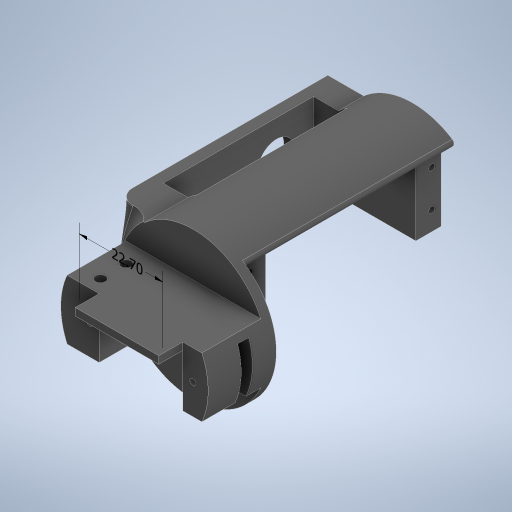
# Autodesk Inventor part: arm_2
Saved by Autodesk Inventor 2024.1 (Build 281209000, 209)
## iProperties
Created: 2025-01-27
Part Number: arm_2
Material: 一般
Document SubType Name: Modeling
Designer: hibik
Density: 1 g/cm^3
Appearance: 既定
Author: hibik
Autodesk Inventor part; units mm, degrees
sketch "スケッチ1" plane through (0, 0, 0) normal (0, 1, 0) x (-1, 0, 0)
  line L0 (11.35, 0) -> (-11.35, 0)
  line L1 (-11.35, 0) -> (-11.35, -25)
  line L2 (-11.35, -25) -> (11.35, -25)
  line L3 (11.35, -25) -> (11.35, 0)
  point P0 (0, 0)
  point P1 (0, 0)
  dimension "d0" = 22.7
  dimension "d9" = 25
  constraints: 8 end point, 2 parallel, 1 coincident, 1 horizontal, 1 midpoint, 1 perpendicular
  measures "d0" distance of L0.start L0.end
  measures "d9" distance of L2.end L0.start
extrude "押し出し1" add sketch "スケッチ1" along normal blind 2
ref_plane "作業平面1" through (-11.35, 0, -22.5) normal (0, 0, 1) x (1, 0, 0)
sketch "スケッチ2" plane through (-11.35, 0, -22.5) normal (0, 0, 1) x (1, 0, 0)
  line L0 (0, 0) -> (0, 2) projected
  line L1 (0, 0) -> (22.7, 0)
  line L2 (22.7, 0) -> (22.7, -12.2)
  line L3 (22.7, -12.2) -> (0, -12.2)
  line L4 (0, -12.2) -> (0, 0)
  line L5 (22.7, 0) -> (22.7, 2) projected
  line L6 (0, -12.2) -> (22.7, -12.2)
  line L7 (22.7, -12.2) -> (22.7, -14.2)
  line L8 (22.7, -14.2) -> (0, -14.2)
  line L9 (0, -14.2) -> (0, -12.2)
  circle A0 centre (9.6, -6.1) radius 20
  line L10 (0, -14.2) -> (-8.6863, -14.2)
  line L11 (-8.6863, -14.2) -> (-8.6863, 2)
  line L12 (-8.6863, 2) -> (0, 2)
  line L13 (0, 2) -> (0, -14.2)
  line L14 (22.7, -14.2) -> (27.8863, -14.2)
  line L15 (27.8863, -14.2) -> (27.8863, 2)
  line L16 (27.8863, 2) -> (22.7, 2)
  line L17 (22.7, 2) -> (22.7, -14.2)
  circle A1 centre (9.6, -6.1) radius 17.5 construction
  circle A2 centre (16.6, -6.1) radius 10.5 construction
  circle A3 centre (16.6, -6.1) radius 6.1
  line L18 (0, 0) -> (22.7, 0) projected
  point P0 (11.35, 0)
  point P1 (22.7, 0)
  dimension "d4" = 12.2
  dimension "d5" = 2
  dimension "d6" = 40
  dimension "d32" = 35
  dimension "d33" = 21
  constraints: 32 end point, 8 parallel, 4 centre point, 4 horizontal, 4 perpendicular, 4 point on circle, 4 tangent, 2 coincident, 2 collinear, 1 horizontal alignment
  measures "d4" distance of L1.end L2.end
  measures "d5" distance of L6.end L7.end
  measures "d6" diameter of A0
  measures "d32" diameter of A1
  measures "d33" diameter of A2
extrude "押し出し2" add sketch "スケッチ2" against normal blind 2.5
ref_plane "作業平面3" through (11.35, 0, -25) normal (0, 0, -1) x (-1, 0, 0)
sketch "スケッチ4" plane through (11.35, 0, -25) normal (0, 0, -1) x (-1, 0, 0)
  line L0 (-0.1288, 8.9) -> (26.3288, 8.9)
  circle A0 centre (13.1, -6.1) radius 20 projected
  line L1 (22.7, 2) -> (0, 2) projected
  dimension "d40" = 15
  constraints: 2 end point, 2 point on circle, 1 horizontal
  measures "d40" distance from line of A0.centre L0
extrude "押し出し4" add sketch "スケッチ4" along normal blind 57 contours A0 L0 picked at (10.0107, 9.8077)
ref_plane "作業平面2" through (7.9, 0, -25) normal (1, 0, 0) x (0, 0, -1)
extrude "押し出し7" add sketch "スケッチ2" along normal blind 16 contours L4 L9 L10 L11 L12 L0 | L11 A0 | L5 L16 L15 L14 L7 L2 | A0 L15
sketch "スケッチ7" plane through (11.35, -14.2, -22.5) normal (0, -1, 0) x (1, 0, 0)
  line L0 (0, 16) -> (0, 0) projected
  line L1 (0, 4) -> (19.8753, 4)
  line L2 (19.8753, 4) -> (19.8753, 7)
  line L3 (19.8753, 7) -> (0, 7)
  line L4 (0, 7) -> (0, 4)
  line L5 (5.1863, 0) -> (-31.3863, 0) projected
  point P0 (-11.35, 22.5)
  point P1 (0, 7)
  dimension "d28" = 4
  dimension "d29" = 3
  constraints: 8 end point, 2 parallel, 1 horizontal, 1 perpendicular, 1 point on line
  measures "d28" distance between parallel lines of L5 L1
  measures "d29" distance of L1.end L2.end
extrude "押し出し8" cut sketch "スケッチ7" against normal up to surface (14.2 mm away)
sketch "スケッチ9" plane through (0, 2, 0) normal (0, 1, 0) x (1, 0, 0)
  circle A0 centre (-14.6932, 17.2) radius 1.6 projected
  circle A1 centre (-14.6932, 10.2) radius 1.6 projected
  circle A2 centre (-14.6932, 17.2) radius 1.35
  circle A3 centre (-14.6932, 10.2) radius 1.35
  point P0 (0, 0)
  dimension "d34" = 2.7
  dimension "d35" = 2.7
  constraints: 2 centre point, 2 coincident
  measures "d34" diameter of A2
  measures "d35" diameter of A3
extrude "押し出し9" cut sketch "スケッチ9" against normal through all contours A2 | A3
ref_plane "作業平面6" through (6.05, -6.1, -22.5) normal (1, 0, 0) x (0, 0, -1)
ref_plane "作業平面5" through (-1.75, -6.1, -22.5) normal (1, 0, 0) x (0, 0, -1)
sketch "スケッチ10" plane through (6.05, -6.1, -22.5) normal (1, 0, 0) x (0, 0, -1)
  line L0 (2.5, 15) -> (59.5, 15) projected
  line L1 (59.5, 15) -> (52.6, 15)
  line L2 (52.6, 15) -> (52.6, -5.1)
  line L3 (52.6, -5.1) -> (59.5, -5.1)
  line L4 (59.5, -5.1) -> (59.5, 15)
  line L5 (2.5, -20) -> (2.5, 15) projected
  line L6 (11.8, 15) -> (2.5, 15)
  line L7 (2.5, 15) -> (2.5, -5.1)
  line L8 (2.5, -5.1) -> (11.8, -5.1)
  line L9 (11.8, -5.1) -> (11.8, 15)
  point P0 (-22.5, 6.1)
  dimension "d43" = 20.1
  dimension "d44" = 40.8
  dimension "d45" = 6.9
  constraints: 16 end point, 4 parallel, 2 horizontal, 2 perpendicular, 2 point on line, 1 collinear
  measures "d43" distance of L3.end L0.end
  measures "d44" distance between parallel lines of L2 L9
  measures "d45" distance of L2.end L3.end
extrude "押し出し10" add sketch "スケッチ10" against normal up to surface round surface about axis through (-1.75, -6.1, -22.5) along (0, 0, -1) radius 20 far side no
fillet "フィレット1" radius 1 2 edges at (11.4788, 8.9, -53.5) (-14.9788, 8.9, -54.7)
ref_plane "作業平面8" through (-24.75, -6.1, -22.5) normal (1, 0, 0) x (0, 0, -1)
ref_plane "作業平面7" through (-26.75, -6.1, -22.5) normal (1, 0, 0) x (0, 0, -1)
sketch "スケッチ11" plane through (-24.75, -6.1, -22.5) normal (1, 0, 0) x (0, 0, -1)
  line L0 (2.5, -20) -> (2.5, 16.8421) projected
  line L1 (59.5, -5.1) -> (59.5, 20) projected
  line L2 (52.6, -5.1) -> (59.5, -5.1) projected
  line L3 (2.5, -5.1) -> (11.8, -5.1) projected
  line L4 (11.8, 15) -> (52.6, 15) projected
  line L5 (59.5, -5.1) -> (2.5, -5.1)
  line L6 (2.5, -5.1) -> (2.5, 15)
  line L7 (2.5, 15) -> (59.5, 15)
  line L8 (59.5, 15) -> (59.5, -5.1)
  point P0 (-22.5, 6.1)
  point P1 (59.5, 16.8421)
  point P2 (59.5, 15)
  constraints: 8 end point, 2 parallel, 1 collinear, 1 horizontal, 1 perpendicular, 1 point on line
extrude "押し出し11" add sketch "スケッチ11" along normal blind 3
sketch "スケッチ12" plane through (-21.75, -6.1, -22.5) normal (1, 0, 0) x (0, 0, -1)
  line L0 (11.8, -5.1) -> (11.8, 15) projected
  line L1 (52.6, 15) -> (52.6, -5.1) projected
  line L2 (59.5, -5.1) -> (59.5, 15) projected
  line L3 (2.5, -20) -> (2.5, 16.8421) projected
  line L4 (59.5, 15) -> (2.5, 15) projected
  line L5 (59.5, -5.1) -> (59.5, 15) projected
  line L6 (2.5, -5.1) -> (59.5, -5.1) projected
  line L7 (2.5, 15) -> (2.5, -5.1) projected
  point P0 (-22.5, 6.1)
  point P1 (11.8, 15)
  point P2 (2.5, 15)
  point P3 (59.5, 15)
extrude "押し出し12" add sketch "スケッチ12" along normal up to surface contours L6 L3 L4 L0 | L1 L4 L2 L6 round surface about axis through (-1.75, -6.1, -22.5) along (0, 0, -1) radius 20 far side no
sketch "スケッチ13" plane through (-24.75, -6.1, -22.5) normal (-1, 0, 0) x (0, 0, 1)
  circle A0 centre (-42.55, 4.95) radius 10.05
  line L0 (-52.6, 15) -> (-11.8, 15) projected
  line L1 (-2.5, -5.1) -> (-59.5, -5.1) projected
  line L2 (-52.6, -5.1) -> (-52.6, 15) projected
  line L3 (-52.6, 15) -> (-52.6, -5.1) projected
  circle A1 centre (-42.55, 4.95) radius 5
  line L4 (-52.6, 16.8421) -> (-52.6, 15) projected
  line L5 (-52.6, 16.8421) -> (-52.6, 15) projected
  point P0 (22.5, 6.1)
  dimension "d55" = 10
  constraints: 3 tangent, 2 centre point, 1 coincident
  measures "d55" diameter of A1
extrude "押し出し13" cut sketch "スケッチ13" against normal up to surface (3 mm away) contours A1
fillet "フィレット2" radius 4 2 edges at (-24.75, -1.15, -25) (-20.8854, -0.2832, -25)
sketch "スケッチ14" plane through (6.05, -6.1, -22.5) normal (1, 0, 0) x (0, 0, -1)
  arc A0 (5.5792, 8.7) -> (5.5792, 11.2) centre (7.45, 9.95) ccw projected
  arc A1 (5.5792, -1.3) -> (5.5792, 1.2) centre (7.45, -0.05) ccw projected
  arc A2 (58.8208, 11.2) -> (58.8208, 8.7) centre (56.95, 9.95) ccw projected
  arc A3 (58.8208, 1.2) -> (58.8208, -1.3) centre (56.95, -0.05) ccw projected
  circle A4 centre (7.45, 9.95) radius 0.85
  circle A5 centre (56.95, 9.95) radius 0.85
  circle A6 centre (56.95, -0.05) radius 0.85
  circle A7 centre (7.45, -0.05) radius 0.85
  point P0 (-22.5, 6.1)
  dimension "d59" = 1.7
  dimension "d60" = 1.7
  dimension "d61" = 1.7
  dimension "d62" = 1.7
  constraints: 4 centre point, 4 coincident
  measures "d59" diameter of A4
  measures "d60" diameter of A5
  measures "d61" diameter of A6
  measures "d62" diameter of A7
extrude "押し出し14" cut sketch "スケッチ14" against normal blind 10
sketch "スケッチ15" plane through (-24.75, -6.1, -22.5) normal (-1, 0, 0) x (0, 0, 1)
  line L0 (-11.8, 15) -> (-11.8, -5.1) projected
  line L1 (-11.8, -5.1) -> (-52.6, -5.1) projected
  line L2 (-11.8, -5.1) -> (-26.8, -5.1)
  line L3 (-26.8, -5.1) -> (-26.8, 2.9)
  line L4 (-26.8, 2.9) -> (-11.8, 2.9)
  line L5 (-11.8, 2.9) -> (-11.8, -5.1)
  point P0 (22.5, 6.1)
  point P1 (-11.8, 2.9)
  point P2 (-26.8, -5.1)
  dimension "d65" = 8
  dimension "d66" = 15
  constraints: 8 end point, 2 parallel, 1 horizontal, 1 perpendicular
  measures "d65" distance between parallel lines of L1 L4
  measures "d66" distance of L3.end L4.end
extrude "押し出し15" cut sketch "スケッチ15" against normal up to surface (3 mm away)
fillet "フィレット3" radius 4 3 edges at (-23.25, -3.2, -49.3) (-23.25, -11.2, -49.3) (-23.25, -3.2, -34.3)
sketch "スケッチ16" plane through (-11.35, 0, -6.5) normal (0, 0, 1) x (1, 0, 0)
  arc A0 (26.316, -5.6) -> (26.316, -6.6) centre (25.45, -6.1) ccw projected
  arc A1 (-3.416, -6.6) -> (-3.416, -5.6) centre (-2.55, -6.1) ccw projected
  circle A2 centre (-2.55, -6.1) radius 0.85
  circle A3 centre (25.45, -6.1) radius 0.85
  point P0 (11.35, 0)
  dimension "d70" = 1.7
  dimension "d71" = 1.7
  constraints: 2 centre point, 2 coincident
  measures "d70" diameter of A2
  measures "d71" diameter of A3
extrude "押し出し16" cut sketch "スケッチ16" against normal blind 10
ref_plane "作業平面4" through (18.25, -6.1, -22.5) normal (1, 0, 0) x (0, 0, -1)
